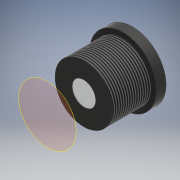
# Autodesk Inventor part: Lens_M12_12.0mm-f2.8
Saved by Autodesk Inventor 2018 (Build 220112000, 112)
## iProperties
Created: 2018-07-29
Part Number: Lens_M12_12.0mm-f2.8
Material: ABS Plastic
Document SubType Name: Modeling
Designer: Bradley
Density: 1.06 g/cm^3
Appearance: Smooth - Black
Description: SVL-IR1228B5M
Author: Bradley
Autodesk Inventor part; units mm, degrees
ref_plane "YZ Plane" through (0, 0, 0) normal (1, 0, 0) x (0, 1, 0)
ref_plane "XZ Plane" through (0, 0, 0) normal (0, 1, 0) x (-1, 0, 0)
ref_plane "XY Plane" through (0, 0, 0) normal (0, 0, 1) x (1, 0, 0)
sketch "Sketch1" plane through (0, 0, 0) normal (0, 0, 1) x (1, 0, 0)
  line L0 (0, 5.05) -> (0, -5.05)
  line L1 (6, -5.15) -> (6, 3.05)
  line L2 (6, 3.05) -> (7, 3.05)
  line L3 (7, 3.05) -> (7, 5.05)
  line L4 (7, 5.05) -> (2.2235, 5.05)
  line L5 (2.2235, 5.05) -> (2.14, 4.8207)
  arc A0 (2.14, 4.8207) -> (0, 5.05) centre (0, -5.05) ccw
  line L6 (0, -12.74) -> (6, -12.74)
  line L7 (0, -5.05) -> (2.5, -5.05)
  line L8 (2.5, -5.05) -> (2.5, -5.15)
  line L9 (2.5, -5.15) -> (6, -5.15)
  point P0 (0, 0)
  point P1 (0, 0)
  dimension "d2" = 12
  dimension "d3" = 14
  dimension "d4" = 2
  dimension "d6" = 110
  dimension "d11" = 5
  dimension "d12" = 7.59
  dimension "d13" = 0.1
  dimension "d14" = 17.79
  dimension "d16" = 10.2
  dimension "d17" = 4.28
  constraints: 20 end point, 5 perpendicular, 2 coincident, 2 horizontal, 2 point on circle, 2 point on line, 1 centre point, 1 line through centre, 1 midpoint, 1 vertical
  measures "d2" diameter of L1 L0
  measures "d3" diameter of L3 L0
  measures "d4" distance of L2.end L3.end
  measures "d6" angle of L4 L5
  measures "d11" diameter of L8 L0
  measures "d12" distance between parallel lines of L6 L9
  measures "d13" distance of L7.end L8.end
  measures "d14" distance from line of L6 L0.start
  measures "d16" distance between parallel lines of L4 L9
  measures "d17" diameter of L5.end L0
revolve "Revolution1" add sketch "Sketch1" angle 360 about axis through (0, 5.05, 0) along (0, -1, 0)
surface revolve "RevolutionSrf1" sketch "Sketch1" angle 360 about axis through (0, 5.05, 0) along (0, -1, 0) shown yes curves L6
thread "Thread1" size "M12x0.5" class "6g" standard "ANSI Metric M Profile" full length
body "Solid1"
body "Srf1"
